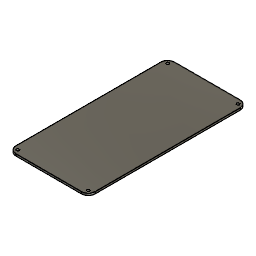
topBoard (Autodesk Fusion 360 design; units mm, degrees)
Autodesk Fusion 360 part; units mm, degrees
note: some values were not read from the file. Set by a fixed rule: which face or edge a step refers to.
sketch "Sketch1" plane through (0, 0, 0) normal (0, 0, 1) x (1, 0, 0)
  line L0 (-50.8, 101.6) -> (50.8, 101.6)
  line L1 (50.8, 101.6) -> (50.8, -101.6)
  line L2 (50.8, -101.6) -> (-50.8, -101.6)
  line L3 (-50.8, -101.6) -> (-50.8, 101.6)
  line L4 (-50.8, 101.6) -> (50.8, -101.6) construction
  line L5 (50.8, 101.6) -> (-50.8, -101.6) construction
  dimension "d1" = 101.6
  dimension "d2" = 203.2
  constraint horizontal L0
  constraint vertical L1
  constraint horizontal L2
  constraint vertical L3
  constraint coincident origin L5
  constraint midpoint origin L4
  measures "d1" distance of L0.start L0.end
  measures "d2" distance of L0.start L2.end
extrude "Extrude1" add sketch "Sketch1" along normal blind 2.54
fillet "Fillet1" radius 8.89 4 edges at (-50.8, -101.6, 1.27) (50.8, -101.6, 1.27) (50.8, 101.6, 1.27) (-50.8, 101.6, 1.27)
sketch "Sketch2" plane through (0, 0, 2.54) normal (0, 0, 1) x (-1, 0, 0)
  arc A0 (41.91, -101.6) -> (50.8, -92.71) centre (41.91, -92.71) ccw
  line L0 (50.8, -92.71) -> (50.8, 92.71)
  arc A1 (50.8, 92.71) -> (41.91, 101.6) centre (41.91, 92.71) ccw
  line L1 (41.91, 101.6) -> (-41.91, 101.6)
  arc A2 (-41.91, 101.6) -> (-50.8, 92.71) centre (-41.91, 92.71) ccw
  line L2 (-50.8, 92.71) -> (-50.8, -92.71)
  arc A3 (-50.8, -92.71) -> (-41.91, -101.6) centre (-41.91, -92.71) ccw
  line L3 (-41.91, -101.6) -> (41.91, -101.6)
  line L4 (41.91, -92.71) -> (-41.91, -92.71) construction
  line L5 (-41.91, -92.71) -> (-41.91, 92.71) construction
  line L6 (-41.91, 92.71) -> (41.91, 92.71) construction
  line L7 (41.91, 92.71) -> (41.91, -92.71) construction
  line L8 (41.91, 92.71) -> (48.1962, 98.9962) construction
  arc A4 (41.91, 101.6) -> (50.8, 92.71) centre (53.2921, 104.0921) ccw construction
  circle A5 centre (45.0531, 95.8531) radius 1.778
  point P0 (45.0531, 95.8531)
  point P1 (46.3103, 97.1103)
  point P2 (43.7959, 94.5959)
  dimension "d7" = 8.89
  dimension "d8" = 8.89
  dimension "d9" = 8.89
  dimension "d10" = 8.89
  dimension "d11" = 185.42
  dimension "d12" = 83.82
  dimension "d13" = 3.556
  constraint horizontal L4
  constraint vertical L5
  constraint horizontal L6
  constraint vertical L7
  constraint coincident A1.centre L6.end
  constraint midpoint A1 L8.end
  constraint midpoint L8 P0
  constraint coincident P0 A4
  constraint coincident A1.end L1.start
  constraint coincident L0.end A1.start
  constraint coincident P0 A5.centre
  constraint coincident A5 P1
  constraint coincident L8 P1
  constraint coincident L8 P2
  constraint coincident A5 P2
  measures "d7" distance of L0 L7
  measures "d8" distance of L2 L5
  measures "d9" distance of L3 L4
  measures "d10" distance of L1 L6
  measures "d11" distance of L4 L6
  measures "d12" distance of A0.centre A3.centre
  measures "d13" diameter of A5
extrude "Extrude3" cut sketch "Sketch2" against normal blind 15 contours A5
mirror "Mirror3" about plane through (0, 0, 0) normal (0, 1, 0) of 1 faces at (-43.4147, -95.1625, 0.8467)
mirror "Mirror4" about plane through (0, 0, 0) normal (1, 0, 0) of 2 faces at (-43.4147, -95.1625, 0.8467) (-43.4147, 95.1625, 0.8467)
extrude "Extrude2" [suppressed]
